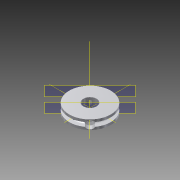
# Autodesk Inventor part: spring_cam
Saved by Autodesk Inventor 2015 (Build 190159000, 159)
## iProperties
Created: 2015-08-29
Part Number: spring_cam
Material: Aluminum 6061
Description: insert part description/title
Document SubType Name: Modeling
Designer: francis
Density: 2.7 g/cm^3
Appearance: Aluminum - Flat
Mass: 5.08251 g
Surface Area: 18.1679 cm^2
Volume: 1.88241 cm^3
Part Category: insert part category here and press enter to fill value
Author: francis
Autodesk Inventor part; units mm, degrees
ref_plane "YZ Plane" through (0, 0, 0) normal (1, 0, 0) x (0, 1, 0)
ref_plane "XY Plane" through (0, 0, 0) normal (0, 0, 1) x (1, 0, 0)
sketch "Sketch1" plane through (0, 0, 0) normal (1, 0, 0) x (0, 1, 0)
  line L0 (0, 2.75) -> (12.5, 2.75)
  line L1 (12.5, 2.75) -> (12.5, 1.25)
  line L2 (-2.5, 0) -> (15, 0) construction
  line L3 (0, -7.196) -> (0, 7.896) construction
  line L4 (0, 2.75) -> (0, 0)
  line L5 (0, 7.196) -> (0, -7.896) construction
  line L6 (0, -2.75) -> (0, 0)
  line L7 (12.5, 1.25) -> (10.5, 1.25)
  arc A0 (10.5, 1.25) -> (9.25, 0) centre (10.5, 0) ccw
  line L8 (0, -2.75) -> (12.5, -2.75)
  line L9 (12.5, -2.75) -> (12.5, -1.25)
  line L10 (0, -2.75) -> (0, 0)
  line L11 (12.5, -1.25) -> (10.5, -1.25)
  arc A1 (9.25, 0) -> (10.5, -1.25) centre (10.5, 0) ccw
  point P0 (10.0857, 0)
  dimension "d0" = 12.5
  dimension "d3" = 1.5
  dimension "d15" = 1.25
  dimension "d16" = 2
  constraints: 20 end point, 6 symmetric about line, 4 point on circle, 4 point on line, 2 centre point, 2 horizontal, 1 line through centre, 1 perpendicular, 1 tangent, 1 vertical, 1 other
  measures "d0" distance of L0.start L0.end
  measures "d3" distance of L0.end L1.end
  measures "d15" radius of A0
  measures "d16" distance of L1.end L7.end
revolve "Revolution1" add sketch "Sketch1" angle 360 about axis through (0, 0, -10) along (0, 0, 1)
hole "Hole1" at (0, 0, -2.75) direction (0, 0, 1) diameter 8 end through all
sketch "Sketch2" plane through (0, 0, 0) normal (0, 1, 0) x (-1, 0, 0)
  circle A0 centre (0, 0) radius 2.5337
  dimension "d14" = 5.0673
  constraints: 1 centre point, 1 coincident
  measures "d14" diameter of A0
hole "Hole2" at (0, 0, 0) direction (0, -1, 0) diameter 2.459 end through all thread size "M3x0.5" class "6H" standard "ISO Metric profile"
ref_plane "Work Plane1" through (0, 0, 0) normal (-0.7071068, 0.7071068, 0) x (0, 0, 1)
sketch "Sketch5" plane through (0, 0, 0) normal (-0.7071068, 0.7071068, 0) x (0, 0, 1)
  point P0 (0, 0)
  point P1 (0, 0)
  point P2 (0, 0)
  constraints: 2 coincident
hole "Hole3" at (0, 0, 0) at (0, 0, 0) direction (-0.7071068, 0.7071068, 0) diameter 2.459 end through all thread size "M3x0.5" class "6H" standard "ISO Metric profile"
ref_plane "Work Plane2" through (-8.8388, 8.8388, 2) normal (-0.7071068, 0.7071068, 0) x (-0.7071068, -0.7071068, 0)
hole "Hole4" at (-8.8388, 8.8388, 0) direction (0.7071068, -0.7071068, 0) diameter 5 depth 3 tip angle 118
mirror "Mirror2" about plane through (0, 0, 0) normal (-0.7071068, 0.7071068, 0) of "Hole3", "Hole4"
body "Solid1"
